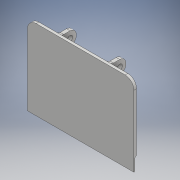
# Autodesk Inventor part: top_right
Saved by Autodesk Inventor 2017 (Build 210142000, 142)
## iProperties
Created: 2017-06-21
Part Number: top_right
Material: Generic
Document SubType Name: Modeling
Designer: erwin
Density: 1 g/cm^3
Appearance: Default
Author: erwin
Autodesk Inventor part; units mm, degrees
ref_plane "YZ Plane" through (0, 0, 0) normal (1, 0, 0) x (0, 1, 0)
ref_plane "XZ Plane" through (0, 0, 0) normal (0, 1, 0) x (-1, 0, 0)
ref_plane "XY Plane" through (0, 0, 0) normal (0, 0, 1) x (1, 0, 0)
sketch "Sketch1" plane through (0, 0, 0) normal (0, 1, 0) x (-1, 0, 0)
  line L0 (0, 0) -> (120, 0)
  line L1 (120, 0) -> (120, 90)
  line L2 (120, 90) -> (0, 90)
  line L3 (0, 90) -> (0, 0)
  dimension "d0" = 120
  dimension "d1" = 90
  constraints: 8 end point, 2 parallel, 1 horizontal, 1 perpendicular
  measures "d0" distance of L2.end L1.end
  measures "d1" distance of L1.end L0.end
extrude "Extrusion1" add sketch "Sketch1" along normal blind 1
fillet "Fillet1" radius 10 2 edges at (-120, 0.5, 90) (0, 0.5, 90)
sketch "Sketch2" plane through (0, 1, 0) normal (0, 1, 0) x (1, 0, 0)
  arc A0 (-10, -90) -> (0, -80) centre (-10, -80) ccw projected
  line L0 (0, -80) -> (0, 0) projected
  line L1 (0, 0) -> (-120, 0) projected
  line L2 (-120, 0) -> (-120, -80) projected
  arc A1 (-120, -80) -> (-110, -90) centre (-110, -80) ccw projected
  line L3 (-110, -90) -> (-10, -90) projected
  arc A2 (-10, -88) -> (-2, -80) centre (-10, -80) ccw
  arc A3 (-118, -80) -> (-110, -88) centre (-110, -80) ccw
  line L4 (-120, 0) -> (-120, -80) projected
  line L5 (0, 0) -> (-120, 0)
  line L6 (-120, 0) -> (-120, -15)
  line L7 (-120, -15) -> (0, -15)
  line L8 (0, -15) -> (0, 0)
  line L9 (0, -15) -> (-120, -15)
  line L10 (-120, -15) -> (-120, -17)
  line L11 (0, -17) -> (0, -15)
  line L12 (-2, -17) -> (-2, -80)
  line L13 (-118, -80) -> (-118, -17)
  line L14 (-60, -17) -> (-60, -88) construction
  line L15 (-87.5, -88) -> (-32.5, -88)
  line L16 (-30, -88) -> (-30, -17)
  line L17 (-32.5, -17) -> (-87.5, -17)
  line L18 (-90, -17) -> (-90, -88)
  line L19 (-87.5, -85.0417) -> (-30, -17) construction
  line L20 (-30, -88) -> (-90, -17) construction
  line L21 (-87.5, -88) -> (-32.5, -88)
  line L22 (-32.5, -88) -> (-32.5, -17)
  line L23 (-32.5, -17) -> (-87.5, -17)
  line L24 (-87.5, -17) -> (-87.5, -88)
  line L25 (-87.5, -88) -> (-32.5, -17) construction
  line L26 (-32.5, -88) -> (-87.5, -17) construction
  line L27 (-10, -88) -> (-30, -88)
  line L28 (-32.5, -88) -> (-87.5, -88)
  line L29 (-90, -88) -> (-110, -88)
  line L30 (-118, -17) -> (-90, -17)
  line L31 (-87.5, -17) -> (-32.5, -17)
  line L32 (-30, -17) -> (-2, -17)
  point P0 (-60, -52.5)
  dimension "d5" = 2
  dimension "d6" = 15
  dimension "d7" = 2
  dimension "d8" = 60
  dimension "d9" = 55
  constraints: 56 end point, 10 parallel, 6 midpoint, 4 horizontal, 4 perpendicular, 4 point on circle, 4 point on line, 2 centre point
  measures "d5" radial gap between concentric circles of A0 A2
  measures "d6" distance of L6.end L5.end
  measures "d7" distance of L10.end L9.end
  measures "d8" distance of L18.start L16.end
  measures "d9" distance of L17.start L17.end
extrude "Extrusion2" add sketch "Sketch2" along normal blind 2 contours L3 A1 L2 L7 L0 A0
fillet "Fillet2" radius 2 1 edges at (-60, 1, 15)
fillet "Fillet3" radius 1 1 edges at (-60, 1, 0)
sketch "Sketch3" plane through (0, 1, 0) normal (0, 1, 0) x (1, 0, 0)
  line L0 (-30, -88) -> (-10, -88) projected
  arc A0 (-10, -88) -> (-2, -80) centre (-10, -80) ccw projected
  line L1 (-2, -80) -> (-2, -17) projected
  line L2 (-2, -17) -> (-30, -17) projected
  line L3 (-30, -17) -> (-30, -88) projected
  line L4 (-32.5, -88) -> (-32.5, -17) projected
  line L5 (-32.5, -17) -> (-87.5, -17) projected
  line L6 (-87.5, -17) -> (-87.5, -88) projected
  line L7 (-87.5, -88) -> (-32.5, -88) projected
  line L8 (-118, -17) -> (-118, -80) projected
  arc A1 (-118, -80) -> (-110, -88) centre (-110, -80) ccw projected
  line L9 (-110, -88) -> (-90, -88) projected
  line L10 (-90, -88) -> (-90, -17) projected
  line L11 (-90, -17) -> (-118, -17) projected
  line L12 (-30, -88) -> (-34, -88)
  line L13 (-34, -88) -> (-34, -73)
  line L14 (-34, -73) -> (-30, -73)
  line L15 (-30, -73) -> (-30, -88)
  line L16 (-90, -88) -> (-86, -88)
  line L17 (-86, -88) -> (-86, -73)
  line L18 (-86, -73) -> (-90, -73)
  line L19 (-90, -73) -> (-90, -88)
  point P0 (0, 0)
  dimension "d14" = 4
  dimension "d15" = 15
  dimension "d16" = 4
  dimension "d17" = 15
  constraints: 16 end point, 4 parallel, 2 horizontal, 2 perpendicular
  measures "d14" distance of L13.end L14.end
  measures "d15" distance of L12.end L13.end
  measures "d16" distance of L18.end L17.end
  measures "d17" distance of L17.end L16.end
extrude "Extrusion3" add sketch "Sketch3" along normal blind 20 contours L12 L4 L14 L3 | L7 L13 L14 L4 | L7 L6 L18 L17 | L16 L10 L18 L6
fillet "Fillet4" radius 7 4 edges at (-32, 21, 73) (-32, 21, 88) (-88, 21, 73) (-88, 21, 88)
fillet "Fillet5" radius 5 2 edges at (-34, 1, 80.5) (-86, 1, 80.5)
sketch "Sketch4" plane through (-90, 1, 17) normal (-1, 0, 0) x (0, 0, 1)
  arc A0 (71, 13) -> (64, 20) centre (64, 13) ccw projected
  line L0 (63, 20) -> (64, 20) projected
  arc A1 (63, 20) -> (56, 13) centre (63, 13) ccw projected
  line L1 (56, 2) -> (56, 13) projected
  line L2 (0, 2) -> (56, 2) projected
  line L3 (0, 0) -> (0, 2) projected
  line L4 (71, 0) -> (0, 0) projected
  line L5 (71, 0) -> (71, 2) projected
  line L6 (71, 2) -> (71, 13) projected
  line L7 (63, 13) -> (64, 13) construction
  point P0 (-17, -1)
  point P1 (63.5, 13)
  constraints: 2 end point, 1 horizontal, 1 midpoint
hole "Hole1" at (-90, 14, 80.5) direction (1, 0, 0) diameter 6 end up to face face through (-30, 6.6667, 78) facing (1, 0, 0)
fillet "Fillet6" radius 5 2 edges at (-87.5, 3, 88) (-32.5, 3, 88)
body "Solid1"
